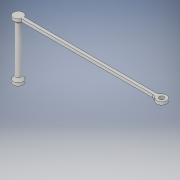
# Autodesk Inventor part: fishing_bar
Saved by Autodesk Inventor 2019 (Build 230136000, 136)
## iProperties
Created: 2020-10-30
Part Number: fishing_bar
Material: Generic
Document SubType Name: Modeling
Designer: Mike
Density: 1 g/cm^3
Appearance: Default
Author: Mike
## iProperties of the stored document fishing_bar_3DPrint.ipt
Created: 2020-11-06
Part Number: fishing_bar_3DPrint
Material: Generic
Document SubType Name: Modeling
Designer: Mike
Density: 1 g/cm^3
Appearance: Default
Author: Mike
Autodesk Inventor part; units mm, degrees
ref_plane "YZ Plane" through (0, 0, 0) normal (1, 0, 0) x (0, 1, 0)
ref_plane "XZ Plane" through (0, 0, 0) normal (0, 1, 0) x (-1, 0, 0)
ref_plane "XY Plane" through (0, 0, 0) normal (0, 0, 1) x (1, 0, 0)
sketch "Sketch1" plane through (0, 0, 0) normal (0, 1, 0) x (-1, 0, 0)
  line L0 (150, 0) -> (150, -3)
  circle A0 centre (-0.077, -1.5638) radius 2.45
  arc A1 (4.6722, 0) -> (4.7123, -3) centre (-0.077, -1.5638) ccw
  line L1 (0, 0) -> (1.809, 0)
  line L2 (4.6722, 0) -> (150, 0)
  line L3 (150, -3) -> (4.7123, -3)
  point P0 (1.809, -3.1277)
  dimension "d0" = 150
  dimension "d1" = 3
  dimension "d2" = 4.9
  dimension "d3" = 10
  constraints: 8 end point, 4 point on circle, 3 perpendicular, 2 centre point, 2 horizontal, 1 coincident
  measures "d0" distance of L1.start L0.start
  measures "d1" distance of L0.start L0.end
  measures "d2" diameter of A0
  measures "d3" diameter of A1
extrude "Extrusion1" add sketch "Sketch1" along normal blind 3
fillet "Fillet1" radius 1 4 edges at (-150, 1.5, 0) (-150, 1.5, -3) (-150, 3, -1.5) (-150, 0, -1.5)
fillet "Fillet2" radius 5 2 edges at (-4.6722, 1.5, 0) (-4.7123, 1.5, -3)
sketch "Sketch2" plane through (0, 3, 0) normal (0, 1, 0) x (1, 0, 0)
  line L0 (-149, 0) -> (-149, 3) projected
  line L1 (-149, 0) -> (-7.4673, 0) projected
  arc A0 (-3.6952, -1.7181) -> (-7.4673, 0) centre (-7.4673, -5) ccw projected
  arc A1 (-3.6952, -1.7181) -> (-3.7498, 4.7819) centre (0.077, 1.5638) ccw projected
  arc A2 (-7.5765, 3) -> (-3.7498, 4.7819) centre (-7.5765, 8) ccw projected
  line L2 (-7.5765, 3) -> (-149, 3) projected
  circle A3 centre (0.077, 1.5638) radius 2.45 projected
  line L3 (-149, 1.5) -> (-148, 1.5)
  point P0 (0, 0)
  dimension "d9" = 1
  constraints: 2 end point, 1 horizontal, 1 midpoint
  measures "d9" distance of L3.start L3.end
hole "Hole1" at (-148, 3, -1.5) direction (0, -1, 0) diameter 1.5 end through all
sketch "Sketch3" plane through (0, 3, 0) normal (0, 1, 0) x (1, 0, 0)
  circle A0 centre (-148, 1.5) radius 0.75 projected
  line L0 (-149, 0) -> (-149, 3) projected
  line L1 (-149, 0) -> (-7.4673, 0) projected
  arc A1 (-3.6952, -1.7181) -> (-7.4673, 0) centre (-7.4673, -5) ccw projected
  arc A2 (-3.6952, -1.7181) -> (-3.7498, 4.7819) centre (0.077, 1.5638) ccw projected
  arc A3 (-7.5765, 3) -> (-3.7498, 4.7819) centre (-7.5765, 8) ccw projected
  line L2 (-7.5765, 3) -> (-149, 3) projected
  circle A4 centre (0.077, 1.5638) radius 2.45 projected
  circle A5 centre (-148, 1.5) radius 5
  circle A6 centre (-148, 1.5) radius 2.45
  point P0 (0, 0)
  dimension "d17" = 4.9
  dimension "d18" = 4.9
  dimension "d19" = 5
  dimension "d20" = 10
  constraints: 2 centre point, 2 coincident
  measures "d17" diameter of A6
  measures "d18" diameter of A4
  measures "d19" radius of A2
  measures "d20" diameter of A5
extrude "Extrusion2" add sketch "Sketch3" against normal up to surface (3 mm away) contours A6 L2 A5 L1 | L1 A5 L2 A6
extrude "Extrusion3" add sketch "Sketch3" against normal blind 60 contours A0 | L1 A6 L2 L0 | L0 L2 A6 L1
sketch "Sketch4" plane through (0, 3, 0) normal (0, 1, 0) x (1, 0, 0)
  arc A0 (-143.2303, 3) -> (-143.2303, 0) centre (-148, 1.5) ccw projected
  line L0 (-143.2303, 0) -> (-7.4673, 0) projected
  arc A1 (-3.6952, -1.7181) -> (-7.4673, 0) centre (-7.4673, -5) ccw projected
  arc A2 (-3.6952, -1.7181) -> (-3.7498, 4.7819) centre (0.077, 1.5638) ccw projected
  arc A3 (-7.5765, 3) -> (-3.7498, 4.7819) centre (-7.5765, 8) ccw projected
  line L1 (-7.5765, 3) -> (-143.2303, 3) projected
  circle A4 centre (0.077, 1.5638) radius 2.45 projected
  line L2 (-148, 1.5) -> (-143.2303, 0)
  line L3 (-148, 1.5) -> (-148, -3.5)
  circle A5 centre (-148, 1.5) radius 5
  point P0 (0, 0)
  constraints: 4 end point, 1 coincident, 1 point on circle, 1 vertical, 1 vertical alignment, 2 other
extrude "Extrusion4" [suppressed]
fillet "Fillet3" [suppressed]
fillet "Fillet4" [suppressed]
sketch "Sketch5" plane through (-148, -57, -1.5) normal (0, -1, 0) x (1, 0, 0)
  circle A0 centre (0, 0) radius 2.45 projected
  circle A1 centre (148.077, -0.0638) radius 2.45 projected
  line L0 (4.7697, -1.5) -> (140.4235, -1.5) projected
  arc A2 (144.2502, -3.2819) -> (140.4235, -1.5) centre (140.4235, -6.5) ccw projected
  arc A3 (144.2502, -3.2819) -> (144.3048, 3.2181) centre (148.077, -0.0638) ccw projected
  arc A4 (140.5327, 1.5) -> (144.3048, 3.2181) centre (140.5327, 6.5) ccw projected
  line L1 (140.5327, 1.5) -> (4.7697, 1.5) projected
  arc A5 (4.7697, 1.5) -> (4.7697, -1.5) centre (0, 0) ccw projected
  circle A6 centre (0, 0) radius 5
  point P0 (148, 1.5)
  constraints: 1 centre point, 1 coincident, 1 concentric
extrude "Extrusion5" add sketch "Sketch5" against normal blind 3 contours A5 A6
chamfer "Chamfer1" distance 2.5 angle 45 2 edges at (-150.45, 0, -1.5) (-150.45, -54, -1.5)
equation "\"d17\" = d18"
equation "\"d20\" = 2 * d19"
body "Solid1"
